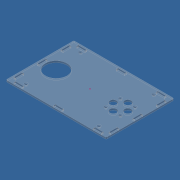
# Autodesk Inventor part: P1704_101
Saved by Autodesk Inventor 2015 (Build 190159000, 159)
## iProperties
Created: 2017-02-08
Part Number: P1704_101
Project: Polymanette chevalier
Material: Plastique PMMA
Description: Toiture
Document SubType Name: Modeling
Designer: Alexandre.PICOTTE
Authority: 185x125.4x3
Density: 1.188 g/cm^3
Appearance: Transparent - Clair
Mass: 73.9833 g
Surface Area: 459.947 cm^2
Volume: 62.2755 cm^3
Material number: ---
Author: Boris.GAUDARD
Autodesk Inventor part; units mm, degrees
ref_plane "Plan YZ" through (0, 0, 0) normal (1, 0, 0) x (0, 1, 0)
ref_plane "Plan XZ" through (0, 0, 0) normal (0, 1, 0) x (-1, 0, 0)
ref_plane "Plan XY" through (0, 0, 0) normal (0, 0, 1) x (1, 0, 0)
sketch "Esquisse1" plane through (0, 0, 0) normal (0, 0, 1) x (1, 0, 0)
  line L0 (-92.5, 62.7) -> (92.5, 62.7)
  line L1 (92.5, 62.7) -> (92.5, -62.7)
  line L2 (92.5, -62.7) -> (-92.5, -62.7)
  line L3 (-92.5, -62.7) -> (-92.5, 62.7)
  line L4 (0, -87.78) -> (0, 87.78) construction
  line L5 (-129.5, 0) -> (129.5, 0) construction
  point P0 (0, 0)
  dimension "d0" = 185
  dimension "d1" = 125.4
  constraints: 8 end point, 2 parallel, 1 horizontal, 1 perpendicular, 2 other
  measures "d0" distance between parallel lines of L1 L3
  measures "d1" distance between parallel lines of L0 L2
extrude "Extrusion1" add sketch "Esquisse1" along normal blind 3
fillet "Congé1" radius 2 4 edges at (-92.5, 62.7, 1.5) (92.5, 62.7, 1.5) (92.5, -62.7, 1.5) (-92.5, -62.7, 1.5)
sketch "Esquisse21" plane through (0, 0, 3) normal (0, 0, 1) x (1, 0, 0)
  line L0 (-129.5, 0) -> (129.5, 0) construction
  line L1 (0, -87.91) -> (0, 88.56) construction
  line L2 (-7.5, 59.7) -> (7.5, 59.7)
  line L3 (7.5, 59.7) -> (7.5, 56.5)
  line L4 (7.5, 56.5) -> (-7.5, 56.5)
  line L5 (-7.5, 56.5) -> (-7.5, 59.7)
  line L6 (-90.5, 62.7) -> (90.5, 62.7) construction
  line L7 (-81, 59.7) -> (-66, 59.7)
  line L8 (-66, 59.7) -> (-66, 56.5)
  line L9 (-66, 56.5) -> (-81, 56.5)
  line L10 (-81, 56.5) -> (-81, 59.7)
  line L11 (-92.5, -60.7) -> (-92.5, 60.7) construction
  line L12 (66, 59.7) -> (81, 59.7)
  line L13 (81, 59.7) -> (81, 56.5)
  line L14 (81, 56.5) -> (66, 56.5)
  line L15 (66, 56.5) -> (66, 59.7)
  line L16 (-81, -56.5) -> (-66, -56.5)
  line L17 (-66, -56.5) -> (-66, -59.7)
  line L18 (-66, -59.7) -> (-81, -59.7)
  line L19 (-81, -59.7) -> (-81, -56.5)
  line L20 (-7.5, -59.7) -> (7.5, -59.7)
  line L21 (7.5, -59.7) -> (7.5, -56.5)
  line L22 (7.5, -56.5) -> (-7.5, -56.5)
  line L23 (-7.5, -56.5) -> (-7.5, -59.7)
  line L24 (66, -59.7) -> (81, -59.7)
  line L25 (81, -59.7) -> (81, -56.5)
  line L26 (81, -56.5) -> (66, -56.5)
  line L27 (66, -56.5) -> (66, -59.7)
  point P0 (0, 0)
  dimension "d216" = 15
  dimension "d217" = 3.2
  dimension "d218" = 3
  dimension "d221" = 11.5
  constraints: 48 end point, 12 parallel, 8 collinear, 6 horizontal, 6 perpendicular, 4 equal length, 1 point on line, 7 other
  measures "d216" distance of L2.start L2.end
  measures "d217" distance of L2.end L3.end
  measures "d218" distance between parallel lines of L6 L2
  measures "d221" distance between parallel lines of L10 L11
extrude "Extrusion8" cut sketch "Esquisse21" against normal through all
sketch "Esquisse24" plane through (0, 0, 3) normal (0, 0, 1) x (1, 0, 0)
  line L0 (-89.5, 7.5) -> (-86.5, 7.5)
  line L1 (-86.5, 7.5) -> (-86.5, -7.5)
  line L2 (-86.5, -7.5) -> (-89.5, -7.5)
  line L3 (-89.5, -7.5) -> (-89.5, 7.5)
  line L4 (86.5, 7.5) -> (89.5, 7.5)
  line L5 (89.5, 7.5) -> (89.5, -7.5)
  line L6 (89.5, -7.5) -> (86.5, -7.5)
  line L7 (86.5, -7.5) -> (86.5, 7.5)
  line L8 (0, -88.56) -> (0, 87.91) construction
  line L9 (-89.5, 51.2) -> (-86.5, 51.2)
  line L10 (-86.5, 51.2) -> (-86.5, 36.2)
  line L11 (-86.5, 36.2) -> (-89.5, 36.2)
  line L12 (-89.5, 36.2) -> (-89.5, 51.2)
  line L13 (-89.5, -36.2) -> (-86.5, -36.2)
  line L14 (-86.5, -36.2) -> (-86.5, -51.2)
  line L15 (-86.5, -51.2) -> (-89.5, -51.2)
  line L16 (-89.5, -51.2) -> (-89.5, -36.2)
  line L17 (89.5, -51.2) -> (86.5, -51.2)
  line L18 (86.5, -51.2) -> (86.5, -36.2)
  line L19 (86.5, -36.2) -> (89.5, -36.2)
  line L20 (89.5, -36.2) -> (89.5, -51.2)
  line L21 (86.5, 51.2) -> (89.5, 51.2)
  line L22 (89.5, 51.2) -> (89.5, 36.2)
  line L23 (89.5, 36.2) -> (86.5, 36.2)
  line L24 (86.5, 36.2) -> (86.5, 51.2)
  line L25 (-92.5, -60.7) -> (-92.5, 60.7) construction
  line L26 (-129.5, 0) -> (129.5, 0) construction
  line L27 (90.5, -62.7) -> (-90.5, -62.7) construction
  point P0 (0, 0)
  dimension "d248" = 15
  dimension "d249" = 3
  dimension "d250" = 3
  dimension "d251" = 11.5
  constraints: 48 end point, 12 parallel, 7 collinear, 6 horizontal, 6 perpendicular, 4 equal length, 4 point on line, 6 other
  measures "d248" distance of L15.end L13.start
  measures "d249" distance of L13.start L13.end
  measures "d250" distance between parallel lines of L25 L16
  measures "d251" distance between parallel lines of L15 L27
extrude "Extrusion9" cut sketch "Esquisse24" against normal through all
sketch "Esquisse23" plane through (0, 0, 3) normal (0, 0, 1) x (1, 0, 0)
  line L0 (0, -87.78) -> (0, 87.78) construction
  line L1 (-129.5, 0) -> (129.5, 0) construction
  point P0 (0, 0)
  point P1 (-67.5, 50.5)
  point P2 (67.5, 50.5)
  point P3 (67.5, -50.5)
  point P4 (-67.5, -50.5)
  dimension "d238" = 135
  dimension "d239" = 101
  constraints: 2 horizontal alignment, 2 symmetric about line, 2 vertical alignment
  measures "d238" distance of point (67.5, 50.5) point (-67.5, 50.5)
  measures "d239" distance of point (-67.5, -50.5) point (-67.5, 50.5)
hole "Perçage11" at (-67.5, 50.5, 3) at (67.5, 50.5, 3) at (67.5, -50.5, 3) at (-67.5, -50.5, 3) direction (0, 0, -1) diameter 3.4 end through all countersink diameter 6.3 countersink angle 90 clearance for "Vis à tête plate fraisée ISO 2009/7046" size "M3" standard "ISO"
sketch "Esquisse19" plane through (0, 0, 3) normal (0, 0, 1) x (1, 0, 0)
  circle A0 centre (-62.5, 0) radius 20
  line L0 (-92.5, -62.7) -> (-92.5, 62.7) construction
  line L1 (92.5, 62.7) -> (92.5, -62.7) construction
  circle A1 centre (43, 0) radius 6.2
  circle A2 centre (56.5, 13.5) radius 6.2
  circle A3 centre (70, 0) radius 6.2
  circle A4 centre (56.5, -13.5) radius 6.2
  line L2 (-129.5, 0) -> (129.5, 0) construction
  line L3 (56.5, 21.3668) -> (56.5, -24.5491) construction
  circle A5 centre (-67.5, -50.5) radius 1.7 construction
  line L4 (86.5, -7.5) -> (86.5, 7.5) projected
  point P0 (0, 0)
  dimension "d178" = 40
  dimension "d193" = 12.4
  dimension "d208" = 27
  dimension "d209" = 27
  dimension "d247" = 5
  dimension "d254" = 16.5
  constraints: 5 centre point, 4 point on line, 3 equal radius, 2 end point, 2 symmetric about line, 1 horizontal alignment, 1 vertical, 1 vertical alignment
  measures "d178" diameter of A0
  measures "d193" diameter of A2
  measures "d208" distance of A1.centre A3.centre
  measures "d209" distance of A4.centre A2.centre
  measures "d247" horizontal distance of A5.centre A0.centre
  measures "d254" distance from line of L4 A3.centre
extrude "Extrusion7" cut sketch "Esquisse19" against normal through all
sketch "Esquisse20" plane through (0, 0, 3) normal (0, 0, 1) x (1, 0, 0)
  line L0 (-129.5, 0) -> (129.5, 0) construction
  circle A0 centre (70, 0) radius 6.2 construction
  circle A1 centre (56.5, 13.5) radius 6.2 construction
  circle A2 centre (43, 0) radius 6.2 construction
  point P0 (0, 0)
  point P1 (43, 13.5)
  point P2 (70, 13.5)
  point P3 (43, -13.5)
  point P4 (70, -13.5)
  constraints: 4 vertical alignment, 3 horizontal alignment, 1 symmetric about line
hole "Perçage8" at (43, 13.5, 3) at (70, 13.5, 3) at (43, -13.5, 3) at (70, -13.5, 3) direction (0, 0, -1) diameter 3.4 end through all countersink diameter 6.3 countersink angle 90 clearance for "Vis à tête plate fraisée ISO 2009/7046" size "M3" standard "ISO"
sketch "Esquisse22" plane through (0, 0, 3) normal (0, 0, 1) x (1, 0, 0)
  line L0 (-81, 59.7) -> (-66, 59.7) construction
  line L1 (-66, 56.5) -> (-81, 56.5) construction
  line L2 (-81, 56.5) -> (-81, 59.7) construction
  line L3 (-66, 59.7) -> (-66, 56.5) construction
  line L4 (-7.5, 56.5) -> (-7.5, 59.7) construction
  line L5 (-7.5, 59.7) -> (7.5, 59.7) construction
  line L6 (7.5, 56.5) -> (-7.5, 56.5) construction
  line L7 (7.5, 59.7) -> (7.5, 56.5) construction
  line L8 (81, 56.5) -> (66, 56.5) construction
  line L9 (66, 59.7) -> (81, 59.7) construction
  line L10 (66, 56.5) -> (66, 59.7) construction
  line L11 (81, 59.7) -> (81, 56.5) construction
  line L12 (7.5, -56.5) -> (7.5, -59.7) construction
  line L13 (7.5, -59.7) -> (-7.5, -59.7) construction
  line L14 (-7.5, -59.7) -> (-7.5, -56.5) construction
  line L15 (-7.5, -56.5) -> (7.5, -56.5) construction
  line L16 (66, 56.5) -> (66, 59.7) construction
  line L17 (66, 59.7) -> (81, 59.7) construction
  line L18 (81, 59.7) -> (81, 56.5) construction
  line L19 (81, 56.5) -> (66, 56.5) construction
  line L20 (-7.5, 56.5) -> (-7.5, 59.7) construction
  line L21 (-7.5, 59.7) -> (7.5, 59.7) construction
  line L22 (7.5, 59.7) -> (7.5, 56.5) construction
  line L23 (7.5, 56.5) -> (-7.5, 56.5) construction
  line L24 (-81, 56.5) -> (-81, 59.7) construction
  line L25 (-81, 59.7) -> (-66, 59.7) construction
  line L26 (-66, 59.7) -> (-66, 56.5) construction
  line L27 (-66, 56.5) -> (-81, 56.5) construction
  line L28 (-81, -59.7) -> (-81, -56.5) construction
  line L29 (-81, -56.5) -> (-66, -56.5) construction
  line L30 (-66, -56.5) -> (-66, -59.7) construction
  line L31 (-66, -59.7) -> (-81, -59.7) construction
  line L32 (81, -56.5) -> (81, -59.7) construction
  line L33 (81, -59.7) -> (66, -59.7) construction
  line L34 (66, -59.7) -> (66, -56.5) construction
  line L35 (66, -56.5) -> (81, -56.5) construction
  circle A0 centre (43, -13.5) radius 3.15 construction
  circle A1 centre (43, 13.5) radius 3.15 construction
  circle A2 centre (70, 13.5) radius 3.15 construction
  circle A3 centre (70, -13.5) radius 3.15 construction
  circle A4 centre (56.5, -13.5) radius 6.2 construction
  circle A5 centre (56.5, 13.5) radius 6.2 construction
  circle A6 centre (43, 0) radius 6.2 construction
  circle A7 centre (70, 0) radius 6.2 construction
  circle A8 centre (-62.5, 0) radius 20 construction
  arc A9 (-92.5, -60.7) -> (-90.5, -62.7) centre (-90.5, -60.7) ccw construction
  line L36 (90.5, -62.7) -> (-90.5, -62.7) construction
  arc A10 (90.5, -62.7) -> (92.5, -60.7) centre (90.5, -60.7) ccw construction
  line L37 (92.5, 60.7) -> (92.5, -60.7) construction
  arc A11 (92.5, 60.7) -> (90.5, 62.7) centre (90.5, 60.7) ccw construction
  line L38 (-90.5, 62.7) -> (90.5, 62.7) construction
  arc A12 (-90.5, 62.7) -> (-92.5, 60.7) centre (-90.5, 60.7) ccw construction
  line L39 (-92.5, -60.7) -> (-92.5, 60.7) construction
  line L40 (-86.5, 51.2) -> (-86.5, 36.2) construction
  line L41 (-89.5, 51.2) -> (-86.5, 51.2) construction
  line L42 (-89.5, 36.2) -> (-89.5, 51.2) construction
  line L43 (-86.5, 36.2) -> (-89.5, 36.2) construction
  line L44 (-86.5, -7.5) -> (-89.5, -7.5) construction
  line L45 (-86.5, 7.5) -> (-86.5, -7.5) construction
  line L46 (-89.5, -7.5) -> (-89.5, 7.5) construction
  line L47 (-89.5, 7.5) -> (-86.5, 7.5) construction
  line L48 (-86.5, -36.2) -> (-86.5, -51.2) construction
  line L49 (-89.5, -36.2) -> (-86.5, -36.2) construction
  line L50 (-89.5, -51.2) -> (-89.5, -36.2) construction
  line L51 (-86.5, -51.2) -> (-89.5, -51.2) construction
  line L52 (89.5, 36.2) -> (86.5, 36.2) construction
  line L53 (86.5, 36.2) -> (86.5, 51.2) construction
  line L54 (86.5, 51.2) -> (89.5, 51.2) construction
  line L55 (89.5, 51.2) -> (89.5, 36.2) construction
  line L56 (86.5, 7.5) -> (89.5, 7.5) construction
  line L57 (86.5, -7.5) -> (86.5, 7.5) construction
  line L58 (89.5, 7.5) -> (89.5, -7.5) construction
  line L59 (89.5, -7.5) -> (86.5, -7.5) construction
  line L60 (86.5, -36.2) -> (89.5, -36.2) construction
  line L61 (86.5, -51.2) -> (86.5, -36.2) construction
  line L62 (89.5, -36.2) -> (89.5, -51.2) construction
  line L63 (89.5, -51.2) -> (86.5, -51.2) construction
  point P0 (0, 0)
  constraints: 24 coincident
hole "Perçage9" at (-81, 59.7, 3) at (-66, 59.7, 3) at (-66, 56.5, 3) at (-81, 56.5, 3) at (-7.5, 59.7, 3) at (7.5, 59.7, 3) at (7.5, 56.5, 3) at (66, 56.5, 3) at (66, 59.7, 3) at (81, 56.5, 3) at (81, 59.7, 3) at (81, -56.5, 3) at (81, -59.7, 3) at (66, -59.7, 3) at (66, -56.5, 3) at (-7.5, -56.5, 3) at (-7.5, -59.7, 3) at (7.5, -59.7, 3) at (-66, -59.7, 3) at (-81, -59.7, 3) at (-7.5, 56.5, 3) at (-81, -56.5, 3) at (-66, -56.5, 3) at (7.5, -56.5, 3) at (-86.5, 51.2, 3) at (-89.5, 51.2, 3) at (-89.5, 36.2, 3) at (-86.5, 36.2, 3) at (-86.5, 7.5, 3) at (-89.5, 7.5, 3) at (-89.5, -7.5, 3) at (-86.5, -7.5, 3) at (-86.5, -36.2, 3) at (-89.5, -36.2, 3) at (-89.5, -51.2, 3) at (-86.5, -51.2, 3) at (86.5, -36.2, 3) at (89.5, -36.2, 3) at (89.5, -51.2, 3) at (86.5, -51.2, 3) at (86.5, -7.5, 3) at (89.5, -7.5, 3) at (86.5, -7.5, 3) at (86.5, 7.5, 3) at (89.5, 7.5, 3) at (86.5, 36.2, 3) at (89.5, 36.2, 3) at (89.5, 51.2, 3) at (86.5, 51.2, 3) direction (0, 0, -1) diameter 1 end through all
sketch "Esquisse25" plane through (0, 0, 3) normal (0, 0, 1) x (1, 0, 0)
  point P0 (0, 0)
